water drip cover_v1 (Autodesk Fusion 360 design; units mm, degrees)
Autodesk Fusion 360 part; units mm, degrees
sketch "Sketch1" plane through (0, 0, 0) normal (1, 0, 0) x (0, 1, 0)
  line L0 (-35, 20) -> (15, 20)
  line L1 (15, 20) -> (15, -30)
  line L2 (15, -30) -> (-35, -30)
  line L3 (-35, -30) -> (-35, 20)
  line L4 (13, -28) -> (-33, -28)
  line L5 (-33, -28) -> (-33, 18)
  line L6 (-33, 18) -> (13, 18)
  line L7 (13, 18) -> (13, -28)
  dimension "d1" = 50
  dimension "d2" = 50
  dimension "d3" = 2
  constraint horizontal L0
  constraint vertical L1
  constraint horizontal L2
  constraint vertical L3
  measures "d1" distance of L0.start L0.end
  measures "d2" distance of L0.start L2.end
extrude "Extrude1" add sketch "Sketch1" along normal blind 2 contours L0 L1 L2 L3 | L4 L5 L6 L7
extrude "Extrude2" add sketch "Sketch1" against normal blind 5
